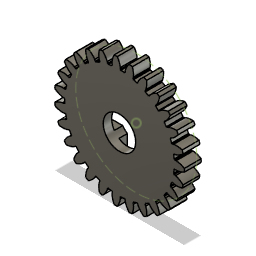
spurGearMaking (Autodesk Fusion 360 design; units mm, degrees)
description: Spur Gear; Module: 0.8; Num Teeth: 27; Pressure Angle: 20.0; Backlash: 0.00 mm
Autodesk Fusion 360 part; units mm, degrees
sketch "Sketch1" plane through (0, 0, 0) normal (0, 0, 1) x (1, 0, 0) in component "Spur Gear (27 teeth)"
  circle A0 centre (0, 0) radius 9.7892
  circle A1 centre (0, 0) radius 2.9
  line L0 (-0.1, 9) -> (0.1, 9)
  line L1 (1.6, 7.5) -> (1.6, -7.5)
  line L2 (0.1, -9) -> (-0.1, -9)
  line L3 (-1.6, -7.5) -> (-1.6, 7.5)
  line L4 (-1.6, 9) -> (1.6, -9) construction
  line L5 (1.6, 9) -> (-1.6, -9) construction
  line L6 (-7, 1.6) -> (7, 1.6)
  line L7 (8.5, 0.1) -> (8.5, -0.1)
  line L8 (7, -1.6) -> (-7, -1.6)
  line L9 (-8.5, -0.1) -> (-8.5, 0.1)
  line L10 (-8.5, 1.6) -> (8.5, -1.6) construction
  line L11 (8.5, 1.6) -> (-8.5, -1.6) construction
  arc A2 (-7, 1.6) -> (-8.5, 0.1) centre (-7, 0.1) ccw
  arc A3 (-8.5, -0.1) -> (-7, -1.6) centre (-7, -0.1) ccw
  arc A4 (8.5, 0.1) -> (7, 1.6) centre (7, 0.1) ccw
  arc A5 (7, -1.6) -> (8.5, -0.1) centre (7, -0.1) ccw
  arc A6 (1.6, 7.5) -> (0.1, 9) centre (0.1, 7.5) ccw
  arc A7 (-0.1, 9) -> (-1.6, 7.5) centre (-0.1, 7.5) ccw
  arc A8 (-1.6, -7.5) -> (-0.1, -9) centre (-0.1, -7.5) ccw
  arc A9 (0.1, -9) -> (1.6, -7.5) centre (0.1, -7.5) ccw
  dimension "d9" = 3.2
  dimension "d10" = 18
  dimension "d11" = 17
  dimension "d12" = 3.2
  dimension "d13" = 1.5
  dimension "d14" = 1.5
  dimension "d15" = 1.5
  dimension "d16" = 1.5
  dimension "d17" = 1.5
  dimension "d18" = 1.5
  dimension "d19" = 1.5
  constraint horizontal L0
  constraint perpendicular L0 L1
  constraint parallel L0 L2
  constraint parallel L1 L3
  constraint coincident L4 A0.centre
  constraint coincident L5 A0.centre
  constraint coincident A0.centre A1.centre
  constraint horizontal L6
  constraint perpendicular L6 L7
  constraint parallel L6 L8
  constraint parallel L7 L9
  constraint coincident L10 A0.centre
  constraint coincident L11 A0.centre
  constraint coincident L10.start L6
  constraint coincident L10.start L9
  constraint tangent L6 A2
  constraint tangent L9 A2
  constraint coincident L11.end L9
  constraint coincident L11.end L8
  constraint tangent L9 A3
  constraint tangent L8 A3
  constraint coincident L11.start L6
  constraint coincident L11.start L7
  constraint tangent L6 A4
  constraint tangent L7 A4
  constraint coincident L10.end L8
  constraint coincident L10.end L7
  constraint tangent L8 A5
  constraint tangent L7 A5
  constraint equal A4 A5
  constraint coincident L5.start L1
  constraint coincident L5.start L0
  constraint tangent L1 A6
  constraint tangent L0 A6
  constraint coincident L4.start L0
  constraint coincident L4.start L3
  constraint tangent L0 A7
  constraint tangent L3 A7
  constraint coincident L5.end L3
  constraint coincident L5.end L2
  constraint tangent L3 A8
  constraint tangent L2 A8
  constraint coincident L4.end L2
  constraint coincident L4.end L1
  constraint tangent L2 A9
  constraint tangent L1 A9
  measures "d9" distance of L4.end L5.end
  measures "d10" distance of L5.start L4.end
  measures "d11" distance of L10.end L11.end
  measures "d12" distance of L11.start L10.end
  measures "d13" radius of A2
  measures "d14" radius of A3
  measures "d15" radius of A4
  measures "d16" radius of A6
  measures "d17" radius of A7
  measures "d18" radius of A8
  measures "d19" radius of A9
extrude "Extrude1" add sketch "Sketch1" along normal blind 3 contours A0 | A1 L6 L7 L8 A4 A5 | A1 L0 L1 L3 A6 A7 | A1 L1 L2 L3 A8 A9 | A1 L6 L8 L9 A2 A3 in component "Spur Gear (27 teeth)"
sketch "Sketch2" plane through (0, 0, 0) normal (0, 0, 1) x (1, 0, 0) in component "Spur Gear (27 teeth)"
  spline S0 degree 5 poles (10.1216, -0.741) (10.1258, -0.7413) (10.1342, -0.7418) (10.1468, -0.7423) (10.1637, -0.7423) (10.1848, -0.7416) (10.2059, -0.7403) (10.2271, -0.7386) (10.2482, -0.7368) (10.2694, -0.7348) (10.2906, -0.7326) (10.3117, -0.7303) (10.3329, -0.7277) (10.3541, -0.7249) (10.3753, -0.7218) (10.3965, -0.7184) (10.4177, -0.7149) (10.4389, -0.7111) (10.4601, -0.7072) (10.4813, -0.7031) (10.5025, -0.6988) (10.5237, -0.6944) (10.5449, -0.6898) (10.5661, -0.6851) (10.5874, -0.6802) (10.6086, -0.6751) (10.6297, -0.6698) (10.6509, -0.6645) (10.6721, -0.6589) (10.6933, -0.6532) (10.7145, -0.6474) (10.7357, -0.6415) (10.7569, -0.6353) (10.778, -0.6291) (10.7992, -0.6227) (10.8204, -0.6162) (10.8415, -0.6096) (10.8627, -0.6028) (10.8838, -0.5959) (10.9049, -0.5888) (10.926, -0.5817) (10.9472, -0.5744) (10.9683, -0.5669) (10.9894, -0.5594) (11.0105, -0.5517) (11.0315, -0.544) (11.0526, -0.536) (11.0737, -0.528) (11.0947, -0.5199) (11.1158, -0.5116) (11.1368, -0.5032) (11.1578, -0.4947) (11.1788, -0.4861) (11.1998, -0.4774) (11.2208, -0.4686) (11.2418, -0.4596) (11.2628, -0.4506) (11.2837, -0.4414) (11.3047, -0.4321) (11.3256, -0.4227) (11.3465, -0.4132) (11.3674, -0.4036) (11.3883, -0.3939) (11.4092, -0.3841) (11.43, -0.3742) (11.4509, -0.3641) (11.4717, -0.354) (11.4925, -0.3438) (11.5133, -0.3334) (11.5341, -0.323) (11.5549, -0.3124) (11.5715, -0.3039) (11.5839, -0.2975) (11.5922, -0.2931) (11.5963, -0.291) knots 0 0 0 0 0 0 0.01428571 0.02857143 0.04285714 0.05714286 0.07142857 0.08571429 0.1 0.11428571 0.12857143 0.14285714 0.15714286 0.17142857 0.18571429 0.2 0.21428571 0.22857143 0.24285714 0.25714286 0.27142857 0.28571429 0.3 0.31428571 0.32857143 0.34285714 0.35714286 0.37142857 0.38571429 0.4 0.41428571 0.42857143 0.44285714 0.45714286 0.47142857 0.48571429 0.5 0.51428571 0.52857143 0.54285714 0.55714286 0.57142857 0.58571429 0.6 0.61428571 0.62857143 0.64285714 0.65714286 0.67142857 0.68571429 0.7 0.71428571 0.72857143 0.74285714 0.75714286 0.77142857 0.78571429 0.8 0.81428571 0.82857143 0.84285714 0.85714286 0.87142857 0.88571429 0.9 0.91428571 0.92857143 0.94285714 0.95714286 0.97142857 0.98571429 1 1 1 1 1 1
  spline S1 degree 5 poles (10.1216, 0.741) (10.1258, 0.7413) (10.1342, 0.7418) (10.1468, 0.7423) (10.1637, 0.7423) (10.1848, 0.7416) (10.2059, 0.7403) (10.2271, 0.7386) (10.2482, 0.7368) (10.2694, 0.7348) (10.2906, 0.7326) (10.3117, 0.7303) (10.3329, 0.7277) (10.3541, 0.7249) (10.3753, 0.7218) (10.3965, 0.7184) (10.4177, 0.7149) (10.4389, 0.7111) (10.4601, 0.7072) (10.4813, 0.7031) (10.5025, 0.6988) (10.5237, 0.6944) (10.5449, 0.6898) (10.5661, 0.6851) (10.5874, 0.6802) (10.6086, 0.6751) (10.6297, 0.6698) (10.6509, 0.6645) (10.6721, 0.6589) (10.6933, 0.6532) (10.7145, 0.6474) (10.7357, 0.6415) (10.7569, 0.6353) (10.778, 0.6291) (10.7992, 0.6227) (10.8204, 0.6162) (10.8415, 0.6096) (10.8627, 0.6028) (10.8838, 0.5959) (10.9049, 0.5888) (10.926, 0.5817) (10.9472, 0.5744) (10.9683, 0.5669) (10.9894, 0.5594) (11.0105, 0.5517) (11.0315, 0.544) (11.0526, 0.536) (11.0737, 0.528) (11.0947, 0.5199) (11.1158, 0.5116) (11.1368, 0.5032) (11.1578, 0.4947) (11.1788, 0.4861) (11.1998, 0.4774) (11.2208, 0.4686) (11.2418, 0.4596) (11.2628, 0.4506) (11.2837, 0.4414) (11.3047, 0.4321) (11.3256, 0.4227) (11.3465, 0.4132) (11.3674, 0.4036) (11.3883, 0.3939) (11.4092, 0.3841) (11.43, 0.3742) (11.4509, 0.3641) (11.4717, 0.354) (11.4925, 0.3438) (11.5133, 0.3334) (11.5341, 0.323) (11.5549, 0.3124) (11.5715, 0.3039) (11.5839, 0.2975) (11.5922, 0.2931) (11.5963, 0.291) knots 0 0 0 0 0 0 0.01428571 0.02857143 0.04285714 0.05714286 0.07142857 0.08571429 0.1 0.11428571 0.12857143 0.14285714 0.15714286 0.17142857 0.18571429 0.2 0.21428571 0.22857143 0.24285714 0.25714286 0.27142857 0.28571429 0.3 0.31428571 0.32857143 0.34285714 0.35714286 0.37142857 0.38571429 0.4 0.41428571 0.42857143 0.44285714 0.45714286 0.47142857 0.48571429 0.5 0.51428571 0.52857143 0.54285714 0.55714286 0.57142857 0.58571429 0.6 0.61428571 0.62857143 0.64285714 0.65714286 0.67142857 0.68571429 0.7 0.71428571 0.72857143 0.74285714 0.75714286 0.77142857 0.78571429 0.8 0.81428571 0.82857143 0.84285714 0.85714286 0.87142857 0.88571429 0.9 0.91428571 0.92857143 0.94285714 0.95714286 0.97142857 0.98571429 1 1 1 1 1 1
  arc A0 (11.5963, -0.291) -> (11.5963, 0.291) centre (0, 0) ccw
  line L0 (9.7531, -0.7148) -> (10.1216, -0.741)
  line L1 (9.7531, 0.7148) -> (10.1216, 0.741)
  line L2 (9.7531, -0.7148) -> (9.7531, 0.7148)
  point P0 (10.2257, -0.7387)
  point P1 (10.3304, -0.728)
  point P2 (10.4354, -0.7117)
  point P3 (10.5407, -0.6907)
  point P4 (10.6462, -0.6656)
  point P5 (10.7518, -0.6368)
  point P6 (10.8575, -0.6044)
  point P7 (10.9633, -0.5687)
  point P8 (11.069, -0.5298)
  point P9 (11.1747, -0.4878)
  point P10 (11.2803, -0.4429)
  point P11 (11.3858, -0.395)
  point P12 (11.4912, -0.3444)
  point P13 (10.2257, 0.7387)
  point P14 (10.3304, 0.728)
  point P15 (10.4354, 0.7117)
  point P16 (10.5407, 0.6907)
  point P17 (10.6462, 0.6656)
  point P18 (10.7518, 0.6368)
  point P19 (10.8575, 0.6044)
  point P20 (10.9633, 0.5687)
  point P21 (11.069, 0.5298)
  point P22 (11.1747, 0.4878)
  point P23 (11.2803, 0.4429)
  point P24 (11.3858, 0.395)
  point P25 (11.4912, 0.3444)
extrude "Extrude2" add sketch "Sketch2" along normal blind 3 in component "Spur Gear (27 teeth)"
fillet "Fillet1" radius 0.1 2 edges at (9.763, -0.7155, 1.5) (9.763, 0.7155, 1.5) in component "Spur Gear (27 teeth)"
pattern_circular "C-Pattern1" count 27 over 360 about axis through (0, 0, 0) along (0, 0, 1) of "Extrude2", "Fillet1" in component "Spur Gear (27 teeth)"
sketch "Sketch3" plane through (0, 0, 0) normal (0, 0, 1) x (1, 0, 0) in component "Spur Gear (27 teeth)"
  circle A0 centre (0, 0) radius 10.8 construction
extrude "Extrude3" cut sketch "Sketch1" along normal blind 1.5 contours A1 L6 L7 L8 A4 A5 | A1 L0 L1 L3 A6 A7 | A1 L1 L2 L3 A8 A9 | A1 L6 L8 L9 A2 A3 in component "Spur Gear (27 teeth)"
component "Spur Gear (27 teeth)" placed x (1, 0, 0) y (0, 1, 0) z (0, 0, 1) at (0, 0, 0)
